Autodesk Inventor part; units mm, degrees
(part 7 of 8)
  spline S913 degree 2 poles (4.9538, -42.7819) (5.0752, -42.7819) (5.2452, -42.6119) (5.2452, -42.4904) knots 0 0 0 1 2 2 2
  line L2980 (4.9538, -42.7819) -> (5.0752, -42.7819) construction
  line L2981 (5.0752, -42.7819) -> (5.2452, -42.6119) construction
  line L2982 (5.2452, -42.6119) -> (5.2452, -42.4904) construction
  line L2983 (5.2452, -42.4904) -> (5.2452, -40.9986)
  spline S914 degree 2 poles (5.2452, -40.9986) (5.2452, -40.8772) (5.0752, -40.7072) (4.9538, -40.7072) knots 0 0 0 1 2 2 2
  line L2984 (5.2452, -40.9986) -> (5.2452, -40.8772) construction
  line L2985 (5.2452, -40.8772) -> (5.0752, -40.7072) construction
  line L2986 (5.0752, -40.7072) -> (4.9538, -40.7072) construction
  line L2987 (4.9538, -40.7072) -> (4.7075, -40.7072)
  spline S915 degree 2 poles (4.7075, -40.7072) (4.5861, -40.7072) (4.4161, -40.8807) (4.4161, -40.9986) knots 0 0 0 1 2 2 2
  line L2988 (4.7075, -40.7072) -> (4.5861, -40.7072) construction
  line L2989 (4.5861, -40.7072) -> (4.4161, -40.8807) construction
  line L2990 (4.4161, -40.8807) -> (4.4161, -40.9986) construction
  line L2991 (4.4161, -40.9986) -> (4.4161, -42.4904)
  spline S916 degree 2 poles (4.4161, -42.4904) (4.4161, -42.6119) (4.5861, -42.7819) (4.7075, -42.7819) knots 0 0 0 1 2 2 2
  line L2992 (4.4161, -42.4904) -> (4.4161, -42.6119) construction
  line L2993 (4.4161, -42.6119) -> (4.5861, -42.7819) construction
  line L2994 (4.5861, -42.7819) -> (4.7075, -42.7819) construction
  line L2995 (4.7075, -42.7819) -> (4.9538, -42.7819)
  spline S917 degree 2 poles (3.9997, -40.9952) (3.9997, -40.7072) (4.4126, -40.2909) (4.7075, -40.2909) knots 0 0 0 1 2 2 2
  line L2996 (3.9997, -40.9952) -> (3.9997, -40.7072) construction
  line L2997 (3.9997, -40.7072) -> (4.4126, -40.2909) construction
  line L2998 (4.4126, -40.2909) -> (4.7075, -40.2909) construction
  line L2999 (4.7075, -40.2909) -> (4.9538, -40.2909)
  spline S918 degree 2 poles (4.9538, -40.2909) (5.2487, -40.2909) (5.6616, -40.7037) (5.6616, -40.9986) knots 0 0 0 1 2 2 2
  line L3000 (4.9538, -40.2909) -> (5.2487, -40.2909) construction
  line L3001 (5.2487, -40.2909) -> (5.6616, -40.7037) construction
  line L3002 (5.6616, -40.7037) -> (5.6616, -40.9986) construction
  line L3003 (5.6616, -40.9986) -> (5.6616, -42.4904)
  spline S919 degree 2 poles (5.6616, -42.4904) (5.6616, -42.7853) (5.2487, -43.1982) (4.9538, -43.1982) knots 0 0 0 1 2 2 2
  line L3004 (5.6616, -42.4904) -> (5.6616, -42.7853) construction
  line L3005 (5.6616, -42.7853) -> (5.2487, -43.1982) construction
  line L3006 (5.2487, -43.1982) -> (4.9538, -43.1982) construction
  line L3007 (4.9538, -43.1982) -> (4.7075, -43.1982)
  spline S920 degree 2 poles (4.7075, -43.1982) (4.4126, -43.1982) (3.9997, -42.7888) (3.9997, -42.4939) knots 0 0 0 1 2 2 2
  line L3008 (4.7075, -43.1982) -> (4.4126, -43.1982) construction
  line L3009 (4.4126, -43.1982) -> (3.9997, -42.7888) construction
  line L3010 (3.9997, -42.7888) -> (3.9997, -42.4939) construction
  spline S921 degree 2 poles (3.5869, -42.99) (3.5869, -43.1982) (3.3787, -43.1982) knots 0 0 0 1 1 1
  line L3011 (3.5869, -42.99) -> (3.5869, -43.1982) construction
  line L3012 (3.5869, -43.1982) -> (3.3787, -43.1982) construction
  spline S922 degree 2 poles (3.3787, -43.1982) (3.1706, -43.1982) (3.1706, -42.99) knots 0 0 0 1 1 1
  line L3013 (3.3787, -43.1982) -> (3.1706, -43.1982) construction
  line L3014 (3.1706, -43.1982) -> (3.1706, -42.99) construction
  line L3015 (3.1706, -42.99) -> (3.1706, -40.499)
  spline S923 degree 2 poles (3.1706, -40.499) (3.1706, -40.2909) (3.3787, -40.2909) knots 0 0 0 1 1 1
  line L3016 (3.1706, -40.499) -> (3.1706, -40.2909) construction
  line L3017 (3.1706, -40.2909) -> (3.3787, -40.2909) construction
  spline S924 degree 2 poles (3.3787, -40.2909) (3.5869, -40.2909) (3.5869, -40.499) knots 0 0 0 1 1 1
  line L3018 (3.3787, -40.2909) -> (3.5869, -40.2909) construction
  line L3019 (3.5869, -40.2909) -> (3.5869, -40.499) construction
  spline S925 degree 2 poles (8.9852, -40.499) (8.9852, -40.2909) (9.1933, -40.2909) knots 0 0 0 1 1 1
  line L3020 (8.9852, -40.499) -> (8.9852, -40.2909) construction
  line L3021 (8.9852, -40.2909) -> (9.1933, -40.2909) construction
  spline S926 degree 2 poles (9.1933, -40.2909) (9.4015, -40.2909) (9.4015, -40.499) knots 0 0 0 1 1 1
  line L3022 (9.1933, -40.2909) -> (9.4015, -40.2909) construction
  line L3023 (9.4015, -40.2909) -> (9.4015, -40.499) construction
  spline S927 degree 2 poles (9.6097, -42.7819) (9.8178, -42.7819) (9.8178, -42.99) knots 0 0 0 1 1 1
  line L3024 (9.6097, -42.7819) -> (9.8178, -42.7819) construction
  line L3025 (9.8178, -42.7819) -> (9.8178, -42.99) construction
  line L3026 (9.8178, -42.99) -> (9.8178, -43.4029)
  spline S928 degree 2 poles (9.8178, -43.4029) (9.8178, -43.611) (9.6097, -43.611) knots 0 0 0 1 1 1
  line L3027 (9.8178, -43.4029) -> (9.8178, -43.611) construction
  line L3028 (9.8178, -43.611) -> (9.6097, -43.611) construction
  spline S929 degree 2 poles (9.6097, -43.611) (9.4015, -43.611) (9.4015, -43.4029) knots 0 0 0 1 1 1
  line L3029 (9.6097, -43.611) -> (9.4015, -43.611) construction
  line L3030 (9.4015, -43.611) -> (9.4015, -43.4029) construction
  spline S930 degree 2 poles (7.3234, -43.1982) (6.9799, -43.1982) (6.4942, -42.7125) (6.4942, -42.369) knots 0 0 0 1 2 2 2
  line L3031 (7.3234, -43.1982) -> (6.9799, -43.1982) construction
  line L3032 (6.9799, -43.1982) -> (6.4942, -42.7125) construction
  line L3033 (6.4942, -42.7125) -> (6.4942, -42.369) construction
  line L3034 (6.4942, -42.369) -> (6.4942, -40.499)
  spline S931 degree 2 poles (6.4942, -40.499) (6.4942, -40.2909) (6.7024, -40.2909) knots 0 0 0 1 1 1
  line L3035 (6.4942, -40.499) -> (6.4942, -40.2909) construction
  line L3036 (6.4942, -40.2909) -> (6.7024, -40.2909) construction
  spline S932 degree 2 poles (6.7024, -40.2909) (6.9105, -40.2909) (6.9105, -40.499) knots 0 0 0 1 1 1
  line L3037 (6.7024, -40.2909) -> (6.9105, -40.2909) construction
  line L3038 (6.9105, -40.2909) -> (6.9105, -40.499) construction
  line L3039 (6.9105, -40.499) -> (6.9105, -42.3655)
  spline S933 degree 2 poles (6.9105, -42.3655) (6.9105, -42.5355) (7.1568, -42.7819) (7.3268, -42.7819) knots 0 0 0 1 2 2 2
  line L3040 (6.9105, -42.3655) -> (6.9105, -42.5355) construction
  line L3041 (6.9105, -42.5355) -> (7.1568, -42.7819) construction
  line L3042 (7.1568, -42.7819) -> (7.3268, -42.7819) construction
  spline S934 degree 2 poles (7.7397, -40.499) (7.7397, -40.2909) (7.9478, -40.2909) knots 0 0 0 1 1 1
  line L3043 (7.7397, -40.499) -> (7.7397, -40.2909) construction
  line L3044 (7.7397, -40.2909) -> (7.9478, -40.2909) construction
  spline S935 degree 2 poles (7.9478, -40.2909) (8.156, -40.2909) (8.156, -40.499) knots 0 0 0 1 1 1
  line L3045 (7.9478, -40.2909) -> (8.156, -40.2909) construction
  line L3046 (8.156, -40.2909) -> (8.156, -40.499) construction
  spline S936 degree 2 poles (-14.1653, -55.9201) (-14.5801, -55.9201) (-15.1811, -55.3275) (-15.1811, -54.9085) knots 0 0 0 1 2 2 2
  line L3047 (-14.1653, -55.9201) -> (-14.5801, -55.9201) construction
  line L3048 (-14.5801, -55.9201) -> (-15.1811, -55.3275) construction
  line L3049 (-15.1811, -55.3275) -> (-15.1811, -54.9085) construction
  line L3050 (-15.1811, -54.9085) -> (-15.1811, -53.3848)
  spline S937 degree 2 poles (-15.1811, -53.3848) (-15.1811, -52.9657) (-14.5801, -52.3732) (-14.1653, -52.3732) knots 0 0 0 1 2 2 2
  line L3051 (-15.1811, -53.3848) -> (-15.1811, -52.9657) construction
  line L3052 (-15.1811, -52.9657) -> (-14.5801, -52.3732) construction
  line L3053 (-14.5801, -52.3732) -> (-14.1653, -52.3732) construction
  line L3054 (-14.1653, -52.3732) -> (-13.4076, -52.3732)
  spline S938 degree 2 poles (-13.4076, -52.3732) (-13.1537, -52.3732) (-13.1537, -52.6271) knots 0 0 0 1 1 1
  line L3055 (-13.4076, -52.3732) -> (-13.1537, -52.3732) construction
  line L3056 (-13.1537, -52.3732) -> (-13.1537, -52.6271) construction
  spline S939 degree 2 poles (-13.1537, -52.6271) (-13.1537, -52.8811) (-13.4076, -52.8811) knots 0 0 0 1 1 1
  line L3057 (-13.1537, -52.6271) -> (-13.1537, -52.8811) construction
  line L3058 (-13.1537, -52.8811) -> (-13.4076, -52.8811) construction
  line L3059 (-13.4076, -52.8811) -> (-14.1653, -52.8811)
  spline S940 degree 2 poles (-14.1653, -52.8811) (-14.3727, -52.8811) (-14.6732, -53.1816) (-14.6732, -53.389) knots 0 0 0 1 2 2 2
  line L3060 (-14.1653, -52.8811) -> (-14.3727, -52.8811) construction
  line L3061 (-14.3727, -52.8811) -> (-14.6732, -53.1816) construction
  line L3062 (-14.6732, -53.1816) -> (-14.6732, -53.389) construction
  line L3063 (-14.6732, -53.389) -> (-14.6732, -54.9043)
  spline S941 degree 2 poles (-14.6732, -54.9043) (-14.6732, -55.1117) (-14.3727, -55.4122) (-14.1653, -55.4122) knots 0 0 0 1 2 2 2
  line L3064 (-14.6732, -54.9043) -> (-14.6732, -55.1117) construction
  line L3065 (-14.6732, -55.1117) -> (-14.3727, -55.4122) construction
  line L3066 (-14.3727, -55.4122) -> (-14.1653, -55.4122) construction
  line L3067 (-14.1653, -55.4122) -> (-13.4076, -55.4122)
  spline S942 degree 2 poles (-13.4076, -55.4122) (-13.1537, -55.4122) (-13.1537, -55.6661) knots 0 0 0 1 1 1
  line L3068 (-13.4076, -55.4122) -> (-13.1537, -55.4122) construction
  line L3069 (-13.1537, -55.4122) -> (-13.1537, -55.6661) construction
  spline S943 degree 2 poles (-13.1537, -55.6661) (-13.1537, -55.9201) (-13.4076, -55.9201) knots 0 0 0 1 1 1
  line L3070 (-13.1537, -55.6661) -> (-13.1537, -55.9201) construction
  line L3071 (-13.1537, -55.9201) -> (-13.4076, -55.9201) construction
  line L3072 (-13.4076, -55.9201) -> (-14.1653, -55.9201)
  spline S944 degree 2 poles (-4.8151, -54.2617) (-5.2315, -54.2617) (-5.2315, -53.8454) knots 0 0 0 1 1 1
  line L3073 (-4.8151, -54.2617) -> (-5.2315, -54.2617) construction
  line L3074 (-5.2315, -54.2617) -> (-5.2315, -53.8454) construction
  spline S945 degree 2 poles (-5.2315, -53.8454) (-5.2315, -53.4291) (-4.8151, -53.4291) knots 0 0 0 1 1 1
  line L3075 (-5.2315, -53.8454) -> (-5.2315, -53.4291) construction
  line L3076 (-5.2315, -53.4291) -> (-4.8151, -53.4291) construction
  line L3077 (-4.8151, -53.4291) -> (-1.4915, -53.4291)
  spline S946 degree 2 poles (-1.4915, -53.4291) (-1.0821, -53.4291) (-1.0821, -53.8454) knots 0 0 0 1 1 1
  line L3078 (-1.4915, -53.4291) -> (-1.0821, -53.4291) construction
  line L3079 (-1.0821, -53.4291) -> (-1.0821, -53.8454) construction
  spline S947 degree 2 poles (-1.0821, -53.8454) (-1.0821, -54.2617) (-1.4915, -54.2617) knots 0 0 0 1 1 1
  line L3080 (-1.0821, -53.8454) -> (-1.0821, -54.2617) construction
  line L3081 (-1.0821, -54.2617) -> (-1.4915, -54.2617) construction
  line L3082 (-1.4915, -54.2617) -> (-4.8151, -54.2617)
  spline S948 degree 2 poles (-18.0718, -61.1463) (-18.0718, -60.9382) (-17.8637, -60.9382) knots 0 0 0 1 1 1
  line L3083 (-18.0718, -61.1463) -> (-18.0718, -60.9382) construction
  line L3084 (-18.0718, -60.9382) -> (-17.8637, -60.9382) construction
  spline S949 degree 2 poles (-17.8637, -60.9382) (-17.6555, -60.9382) (-17.6555, -61.1463) knots 0 0 0 1 1 1
  line L3085 (-17.8637, -60.9382) -> (-17.6555, -60.9382) construction
  line L3086 (-17.6555, -60.9382) -> (-17.6555, -61.1463) construction
  line L3087 (-17.6555, -61.1463) -> (-17.6555, -63.6373)
  spline S950 degree 2 poles (-17.6555, -63.6373) (-17.6555, -63.8455) (-17.8637, -63.8455) knots 0 0 0 1 1 1
  line L3088 (-17.6555, -63.6373) -> (-17.6555, -63.8455) construction
  line L3089 (-17.6555, -63.8455) -> (-17.8637, -63.8455) construction
  spline S951 degree 2 poles (-17.8637, -63.8455) (-18.0718, -63.8455) (-18.0718, -63.6373) knots 0 0 0 1 1 1
  line L3090 (-17.8637, -63.8455) -> (-18.0718, -63.8455) construction
  line L3091 (-18.0718, -63.8455) -> (-18.0718, -63.6373) construction
  spline S952 degree 2 poles (-19.3139, -63.6373) (-19.3139, -63.8455) (-19.522, -63.8455) knots 0 0 0 1 1 1
  line L3092 (-19.3139, -63.6373) -> (-19.3139, -63.8455) construction
  line L3093 (-19.3139, -63.8455) -> (-19.522, -63.8455) construction
  spline S953 degree 2 poles (-19.522, -63.8455) (-19.7302, -63.8455) (-19.7302, -63.6373) knots 0 0 0 1 1 1
  line L3094 (-19.522, -63.8455) -> (-19.7302, -63.8455) construction
  line L3095 (-19.7302, -63.8455) -> (-19.7302, -63.6373) construction
  line L3096 (-19.7302, -63.6373) -> (-19.7302, -61.1463)
  spline S954 degree 2 poles (-19.7302, -61.1463) (-19.7302, -60.9382) (-19.522, -60.9382) knots 0 0 0 1 1 1
  line L3097 (-19.7302, -61.1463) -> (-19.7302, -60.9382) construction
  line L3098 (-19.7302, -60.9382) -> (-19.522, -60.9382) construction
  spline S955 degree 2 poles (-19.522, -60.9382) (-19.3139, -60.9382) (-19.3139, -61.1463) knots 0 0 0 1 1 1
  line L3099 (-19.522, -60.9382) -> (-19.3139, -60.9382) construction
  line L3100 (-19.3139, -60.9382) -> (-19.3139, -61.1463) construction
  spline S956 degree 2 poles (-9.1418, -63.8455) (-9.3499, -63.8455) (-9.3499, -63.6373) knots 0 0 0 1 1 1
  line L3101 (-9.1418, -63.8455) -> (-9.3499, -63.8455) construction
  line L3102 (-9.3499, -63.8455) -> (-9.3499, -63.6373) construction
  spline S957 degree 2 poles (-10.6058, -63.7032) (-10.6509, -63.8455) (-10.7897, -63.8455) knots 0 0 0 1 1 1
  line L3103 (-10.6058, -63.7032) -> (-10.6509, -63.8455) construction
  line L3104 (-10.6509, -63.8455) -> (-10.7897, -63.8455) construction
  spline S958 degree 2 poles (-10.7897, -63.8455) (-11.0083, -63.8455) (-11.0083, -63.6477) knots 0 0 0 1 1 1
  line L3105 (-10.7897, -63.8455) -> (-11.0083, -63.8455) construction
  line L3106 (-11.0083, -63.8455) -> (-11.0083, -63.6477) construction
  spline S959 degree 2 poles (-11.0083, -63.6477) (-11.0083, -63.6096) (-10.9944, -63.5714) knots 0 0 0 1 1 1
  line L3107 (-11.0083, -63.6477) -> (-11.0083, -63.6096) construction
  line L3108 (-11.0083, -63.6096) -> (-10.9944, -63.5714) construction
  line L3109 (-10.9944, -63.5714) -> (-10.1722, -61.0804)
  spline S960 degree 2 poles (-10.1722, -61.0804) (-10.1271, -60.9382) (-9.9779, -60.9382) knots 0 0 0 1 1 1
  line L3110 (-10.1722, -61.0804) -> (-10.1271, -60.9382) construction
  line L3111 (-10.1271, -60.9382) -> (-9.9779, -60.9382) construction
  line L3112 (-9.9779, -60.9382) -> (-9.1418, -60.9382)
  spline S961 degree 2 poles (-9.1418, -60.9382) (-8.9336, -60.9382) (-8.9336, -61.1463) knots 0 0 0 1 1 1
  line L3113 (-9.1418, -60.9382) -> (-8.9336, -60.9382) construction
  line L3114 (-8.9336, -60.9382) -> (-8.9336, -61.1463) construction
  line L3115 (-8.9336, -61.1463) -> (-8.9336, -63.6373)
  spline S962 degree 2 poles (-8.9336, -63.6373) (-8.9336, -63.8455) (-9.1418, -63.8455) knots 0 0 0 1 1 1
  line L3116 (-8.9336, -63.6373) -> (-8.9336, -63.8455) construction
  line L3117 (-8.9336, -63.8455) -> (-9.1418, -63.8455) construction
  spline S963 degree 2 poles (1.8629, -61.1463) (1.8629, -60.9382) (2.0711, -60.9382) knots 0 0 0 1 1 1
  line L3118 (1.8629, -61.1463) -> (1.8629, -60.9382) construction
  line L3119 (1.8629, -60.9382) -> (2.0711, -60.9382) construction
  spline S964 degree 2 poles (2.0711, -60.9382) (2.2793, -60.9382) (2.2793, -61.1463) knots 0 0 0 1 1 1
  line L3120 (2.0711, -60.9382) -> (2.2793, -60.9382) construction
  line L3121 (2.2793, -60.9382) -> (2.2793, -61.1463) construction
  line L3122 (2.2793, -61.1463) -> (2.2793, -63.6373)
  spline S965 degree 2 poles (2.2793, -63.6373) (2.2793, -63.8455) (2.0711, -63.8455) knots 0 0 0 1 1 1
  line L3123 (2.2793, -63.6373) -> (2.2793, -63.8455) construction
  line L3124 (2.2793, -63.8455) -> (2.0711, -63.8455) construction
  spline S966 degree 2 poles (2.0711, -63.8455) (1.8629, -63.8455) (1.8629, -63.6373) knots 0 0 0 1 1 1
  line L3125 (2.0711, -63.8455) -> (1.8629, -63.8455) construction
  line L3126 (1.8629, -63.8455) -> (1.8629, -63.6373) construction
  spline S967 degree 2 poles (0.6209, -63.6373) (0.6209, -63.8455) (0.4128, -63.8455) knots 0 0 0 1 1 1
  line L3127 (0.6209, -63.6373) -> (0.6209, -63.8455) construction
  line L3128 (0.6209, -63.8455) -> (0.4128, -63.8455) construction
  spline S968 degree 2 poles (0.4128, -63.8455) (0.2046, -63.8455) (0.2046, -63.6373) knots 0 0 0 1 1 1
  line L3129 (0.4128, -63.8455) -> (0.2046, -63.8455) construction
  line L3130 (0.2046, -63.8455) -> (0.2046, -63.6373) construction
  line L3131 (0.2046, -63.6373) -> (0.2046, -61.1463)
  spline S969 degree 2 poles (0.2046, -61.1463) (0.2046, -60.9382) (0.4128, -60.9382) knots 0 0 0 1 1 1
  line L3132 (0.2046, -61.1463) -> (0.2046, -60.9382) construction
  line L3133 (0.2046, -60.9382) -> (0.4128, -60.9382) construction
  spline S970 degree 2 poles (0.4128, -60.9382) (0.6209, -60.9382) (0.6209, -61.1463) knots 0 0 0 1 1 1
  line L3134 (0.4128, -60.9382) -> (0.6209, -60.9382) construction
  line L3135 (0.6209, -60.9382) -> (0.6209, -61.1463) construction
  spline S971 degree 2 poles (10.172, -63.4292) (10.342, -63.4292) (10.5848, -63.1828) (10.5848, -63.0128) knots 0 0 0 1 2 2 2
  line L3136 (10.172, -63.4292) -> (10.342, -63.4292) construction
  line L3137 (10.342, -63.4292) -> (10.5848, -63.1828) construction
  line L3138 (10.5848, -63.1828) -> (10.5848, -63.0128) construction
  line L3139 (10.5848, -63.0128) -> (10.5848, -61.7708)
  spline S972 degree 2 poles (10.5848, -61.7708) (10.5848, -61.6008) (10.342, -61.3545) (10.172, -61.3545) knots 0 0 0 1 2 2 2
  line L3140 (10.5848, -61.7708) -> (10.5848, -61.6008) construction
  line L3141 (10.5848, -61.6008) -> (10.342, -61.3545) construction
  line L3142 (10.342, -61.3545) -> (10.172, -61.3545) construction
  spline S973 degree 2 poles (9.3428, -64.8828) (9.3428, -65.091) (9.1347, -65.091) knots 0 0 0 1 1 1
  line L3143 (9.3428, -64.8828) -> (9.3428, -65.091) construction
  line L3144 (9.3428, -65.091) -> (9.1347, -65.091) construction
  spline S974 degree 2 poles (9.1347, -65.091) (8.9265, -65.091) (8.9265, -64.8828) knots 0 0 0 1 1 1
  line L3145 (9.1347, -65.091) -> (8.9265, -65.091) construction
  line L3146 (8.9265, -65.091) -> (8.9265, -64.8828) construction
  line L3147 (8.9265, -64.8828) -> (8.9265, -61.1463)
  spline S975 degree 2 poles (8.9265, -61.1463) (8.9265, -60.9382) (9.1347, -60.9382) knots 0 0 0 1 1 1
  line L3148 (8.9265, -61.1463) -> (8.9265, -60.9382) construction
  line L3149 (8.9265, -60.9382) -> (9.1347, -60.9382) construction
  line L3150 (9.1347, -60.9382) -> (10.172, -60.9382)
  spline S976 degree 2 poles (10.172, -60.9382) (10.5155, -60.9382) (11.0012, -61.4239) (11.0012, -61.7674) knots 0 0 0 1 2 2 2
  line L3151 (10.172, -60.9382) -> (10.5155, -60.9382) construction
  line L3152 (10.5155, -60.9382) -> (11.0012, -61.4239) construction
  line L3153 (11.0012, -61.4239) -> (11.0012, -61.7674) construction
  line L3154 (11.0012, -61.7674) -> (11.0012, -63.0163)
  spline S977 degree 2 poles (11.0012, -63.0163) (11.0012, -63.3598) (10.5155, -63.8455) (10.172, -63.8455) knots 0 0 0 1 2 2 2
  line L3155 (11.0012, -63.0163) -> (11.0012, -63.3598) construction
  line L3156 (11.0012, -63.3598) -> (10.5155, -63.8455) construction
  line L3157 (10.5155, -63.8455) -> (10.172, -63.8455) construction
  spline S978 degree 2 poles (13.0793, -63.4292) (13.2493, -63.4292) (13.4921, -63.1828) (13.4921, -63.0128) knots 0 0 0 1 2 2 2
  line L3158 (13.0793, -63.4292) -> (13.2493, -63.4292) construction
  line L3159 (13.2493, -63.4292) -> (13.4921, -63.1828) construction
  line L3160 (13.4921, -63.1828) -> (13.4921, -63.0128) construction
  spline S979 degree 2 poles (12.663, -61.3545) (12.493, -61.3545) (12.2501, -61.6008) (12.2501, -61.7708) knots 0 0 0 1 2 2 2
  line L3161 (12.663, -61.3545) -> (12.493, -61.3545) construction
  line L3162 (12.493, -61.3545) -> (12.2501, -61.6008) construction
  line L3163 (12.2501, -61.6008) -> (12.2501, -61.7708) construction
  line L3164 (12.2501, -61.7708) -> (12.2501, -63.0128)
  spline S980 degree 2 poles (12.2501, -63.0128) (12.2501, -63.1828) (12.493, -63.4292) (12.663, -63.4292) knots 0 0 0 1 2 2 2
  line L3165 (12.2501, -63.0128) -> (12.2501, -63.1828) construction
  line L3166 (12.2501, -63.1828) -> (12.493, -63.4292) construction
  line L3167 (12.493, -63.4292) -> (12.663, -63.4292) construction
  line L3168 (12.663, -63.4292) -> (13.0793, -63.4292)
  line L3169 (13.0793, -63.8455) -> (12.663, -63.8455)
  spline S981 degree 2 poles (12.663, -63.8455) (12.323, -63.8455) (11.8338, -63.3598) (11.8338, -63.0163) knots 0 0 0 1 2 2 2
  line L3170 (12.663, -63.8455) -> (12.323, -63.8455) construction
  line L3171 (12.323, -63.8455) -> (11.8338, -63.3598) construction
  line L3172 (11.8338, -63.3598) -> (11.8338, -63.0163) construction
  line L3173 (11.8338, -63.0163) -> (11.8338, -61.7674)
  spline S982 degree 2 poles (11.8338, -61.7674) (11.8338, -61.4239) (12.323, -60.9382) (12.663, -60.9382) knots 0 0 0 1 2 2 2
  line L3174 (11.8338, -61.7674) -> (11.8338, -61.4239) construction
  line L3175 (11.8338, -61.4239) -> (12.323, -60.9382) construction
  line L3176 (12.323, -60.9382) -> (12.663, -60.9382) construction
  line L3177 (12.663, -60.9382) -> (13.7003, -60.9382)
  spline S983 degree 2 poles (13.7003, -60.9382) (13.9085, -60.9382) (13.9085, -61.1463) knots 0 0 0 1 1 1
  line L3178 (13.7003, -60.9382) -> (13.9085, -60.9382) construction
  line L3179 (13.9085, -60.9382) -> (13.9085, -61.1463) construction
  line L3180 (13.9085, -61.1463) -> (13.9085, -63.0094)
  spline S984 degree 2 poles (13.9085, -63.0094) (13.9085, -63.3216) (14.1999, -63.4465) knots 0 0 0 1 1 1
  line L3181 (13.9085, -63.0094) -> (13.9085, -63.3216) construction
  line L3182 (13.9085, -63.3216) -> (14.1999, -63.4465) construction
  spline S985 degree 2 poles (14.1999, -63.4465) (14.3283, -63.4985) (14.3283, -63.6304) knots 0 0 0 1 1 1
  line L3183 (14.1999, -63.4465) -> (14.3283, -63.4985) construction
  line L3184 (14.3283, -63.4985) -> (14.3283, -63.6304) construction
  spline S986 degree 2 poles (14.3283, -63.6304) (14.3283, -63.7171) (14.2103, -63.849) (14.1236, -63.849) knots 0 0 0 1 2 2 2
  line L3185 (14.3283, -63.6304) -> (14.3283, -63.7171) construction
  line L3186 (14.3283, -63.7171) -> (14.2103, -63.849) construction
  line L3187 (14.2103, -63.849) -> (14.1236, -63.849) construction
  spline S987 degree 2 poles (14.1236, -63.849) (14.0785, -63.849) (14.0334, -63.8281) knots 0 0 0 1 1 1
  line L3188 (14.1236, -63.849) -> (14.0785, -63.849) construction
  line L3189 (14.0785, -63.849) -> (14.0334, -63.8281) construction
  spline S988 degree 2 poles (14.0334, -63.8281) (13.8252, -63.7379) (13.6968, -63.5714) knots 0 0 0 1 1 1
  line L3190 (14.0334, -63.8281) -> (13.8252, -63.7379) construction
  line L3191 (13.8252, -63.7379) -> (13.6968, -63.5714) construction
  spline S989 degree 2 poles (13.6968, -63.5714) (13.447, -63.8455) (13.0793, -63.8455) knots 0 0 0 1 1 1
  line L3192 (13.6968, -63.5714) -> (13.447, -63.8455) construction
  line L3193 (13.447, -63.8455) -> (13.0793, -63.8455) construction
  line L3194 (15.1574, -60.4386) -> (15.1574, -61.0839)
  spline S990 degree 2 poles (15.1574, -61.0839) (15.3205, -60.9798) (15.5703, -60.7959) knots 0 0 0 1 1 1
  line L3195 (15.1574, -61.0839) -> (15.3205, -60.9798) construction
  line L3196 (15.3205, -60.9798) -> (15.5703, -60.7959) construction
  spline S991 degree 2 poles (15.5703, -60.7959) (15.8201, -60.5947) (15.8201, -60.4386) knots 0 0 0 1 1 1
  line L3197 (15.5703, -60.7959) -> (15.8201, -60.5947) construction
  line L3198 (15.8201, -60.5947) -> (15.8201, -60.4386) construction
  spline S992 degree 2 poles (15.8201, -60.4386) (15.8201, -60.279) (15.716, -60.1888) knots 0 0 0 1 1 1
  line L3199 (15.8201, -60.4386) -> (15.8201, -60.279) construction
  line L3200 (15.8201, -60.279) -> (15.716, -60.1888) construction
  spline S993 degree 2 poles (15.716, -60.1888) (15.6223, -60.109) (15.4905, -60.109) knots 0 0 0 1 1 1
  line L3201 (15.716, -60.1888) -> (15.6223, -60.109) construction
  line L3202 (15.6223, -60.109) -> (15.4905, -60.109) construction
  spline S994 degree 2 poles (15.4905, -60.109) (15.3517, -60.109) (15.2615, -60.1888) knots 0 0 0 1 1 1
  line L3203 (15.4905, -60.109) -> (15.3517, -60.109) construction
  line L3204 (15.3517, -60.109) -> (15.2615, -60.1888) construction
  spline S995 degree 2 poles (15.2615, -60.1888) (15.1574, -60.279) (15.1574, -60.4386) knots 0 0 0 1 1 1
  line L3205 (15.2615, -60.1888) -> (15.1574, -60.279) construction
  line L3206 (15.1574, -60.279) -> (15.1574, -60.4386) construction
  spline S996 degree 2 poles (15.9866, -63.4292) (16.1566, -63.4292) (16.3994, -63.1828) (16.3994, -63.0128) knots 0 0 0 1 2 2 2
  line L3207 (15.9866, -63.4292) -> (16.1566, -63.4292) construction
  line L3208 (16.1566, -63.4292) -> (16.3994, -63.1828) construction
  line L3209 (16.3994, -63.1828) -> (16.3994, -63.0128) construction
  line L3210 (16.3994, -63.0128) -> (16.3994, -61.7674)
  spline S997 degree 2 poles (16.3994, -61.7674) (16.3994, -61.5974) (16.1566, -61.351) (15.9866, -61.351) knots 0 0 0 1 2 2 2
  line L3211 (16.3994, -61.7674) -> (16.3994, -61.5974) construction
  line L3212 (16.3994, -61.5974) -> (16.1566, -61.351) construction
  line L3213 (16.1566, -61.351) -> (15.9866, -61.351) construction
  line L3214 (15.9866, -61.351) -> (15.5703, -61.351)
  spline S998 degree 2 poles (15.5703, -61.351) (15.4003, -61.351) (15.1574, -61.5974) (15.1574, -61.7674) knots 0 0 0 1 2 2 2
  line L3215 (15.5703, -61.351) -> (15.4003, -61.351) construction
  line L3216 (15.4003, -61.351) -> (15.1574, -61.5974) construction
  line L3217 (15.1574, -61.5974) -> (15.1574, -61.7674) construction
  line L3218 (15.1574, -61.7674) -> (15.1574, -63.0128)
  spline S999 degree 2 poles (15.1574, -63.0128) (15.1574, -63.1828) (15.4003, -63.4292) (15.5703, -63.4292) knots 0 0 0 1 2 2 2
  line L3219 (15.1574, -63.0128) -> (15.1574, -63.1828) construction
  line L3220 (15.1574, -63.1828) -> (15.4003, -63.4292) construction
  line L3221 (15.4003, -63.4292) -> (15.5703, -63.4292) construction
  line L3222 (15.5703, -63.4292) -> (15.9866, -63.4292)
  spline S1000 degree 2 poles (16.6111, -61.188) (16.8158, -61.4065) (16.8158, -61.7674) knots 0 0 0 1 1 1
  line L3223 (16.6111, -61.188) -> (16.8158, -61.4065) construction
  line L3224 (16.8158, -61.4065) -> (16.8158, -61.7674) construction
  line L3225 (16.8158, -61.7674) -> (16.8158, -63.0163)
  spline S1001 degree 2 poles (16.8158, -63.0163) (16.8158, -63.3598) (16.3301, -63.8455) (15.9866, -63.8455) knots 0 0 0 1 2 2 2
  line L3226 (16.8158, -63.0163) -> (16.8158, -63.3598) construction
  line L3227 (16.8158, -63.3598) -> (16.3301, -63.8455) construction
  line L3228 (16.3301, -63.8455) -> (15.9866, -63.8455) construction
  line L3229 (15.9866, -63.8455) -> (15.5703, -63.8455)
  spline S1002 degree 2 poles (15.5703, -63.8455) (15.2303, -63.8455) (14.7411, -63.3598) (14.7411, -63.0163) knots 0 0 0 1 2 2 2
  line L3230 (15.5703, -63.8455) -> (15.2303, -63.8455) construction
  line L3231 (15.2303, -63.8455) -> (14.7411, -63.3598) construction
  line L3232 (14.7411, -63.3598) -> (14.7411, -63.0163) construction
  line L3233 (14.7411, -63.0163) -> (14.7411, -60.4386)
  spline S1003 degree 2 poles (14.7411, -60.4386) (14.7411, -60.0882) (14.9735, -59.88) knots 0 0 0 1 1 1
  line L3234 (14.7411, -60.4386) -> (14.7411, -60.0882) construction
  line L3235 (14.7411, -60.0882) -> (14.9735, -59.88) construction
  spline S1004 degree 2 poles (14.9735, -59.88) (15.1852, -59.6927) (15.4939, -59.6927) knots 0 0 0 1 1 1
  line L3236 (14.9735, -59.88) -> (15.1852, -59.6927) construction
  line L3237 (15.1852, -59.6927) -> (15.4939, -59.6927) construction
  spline S1005 degree 2 poles (15.4939, -59.6927) (15.7958, -59.6927) (16.0039, -59.8766) knots 0 0 0 1 1 1
  line L3238 (15.4939, -59.6927) -> (15.7958, -59.6927) construction
  line L3239 (15.7958, -59.6927) -> (16.0039, -59.8766) construction
  spline S1006 degree 2 poles (16.0039, -59.8766) (16.2364, -60.0847) (16.2364, -60.4351) knots 0 0 0 1 1 1
  line L3240 (16.0039, -59.8766) -> (16.2364, -60.0847) construction
  line L3241 (16.2364, -60.0847) -> (16.2364, -60.4351) construction
  spline S1007 degree 2 poles (16.2364, -60.4351) (16.2364, -60.7855) (15.9866, -60.9521) knots 0 0 0 1 1 1
  line L3242 (16.2364, -60.4351) -> (16.2364, -60.7855) construction
  line L3243 (16.2364, -60.7855) -> (15.9866, -60.9521) construction
  spline S1008 degree 2 poles (15.9866, -60.9521) (16.389, -60.9521) (16.6111, -61.188) knots 0 0 0 1 1 1
  line L3244 (15.9866, -60.9521) -> (16.389, -60.9521) construction
  line L3245 (16.389, -60.9521) -> (16.6111, -61.188) construction
  spline S1009 degree 2 poles (20.7639, -63.4292) (20.972, -63.4292) (20.972, -63.6373) knots 0 0 0 1 1 1
  line L3246 (20.7639, -63.4292) -> (20.972, -63.4292) construction
  line L3247 (20.972, -63.4292) -> (20.972, -63.6373) construction
  spline S1010 degree 2 poles (20.972, -63.6373) (20.972, -63.8455) (20.7639, -63.8455) knots 0 0 0 1 1 1
  line L3248 (20.972, -63.6373) -> (20.972, -63.8455) construction
  line L3249 (20.972, -63.8455) -> (20.7639, -63.8455) construction
  spline S1011 degree 2 poles (20.7639, -63.8455) (20.5557, -63.8455) (20.5557, -63.6373) knots 0 0 0 1 1 1
  line L3250 (20.7639, -63.8455) -> (20.5557, -63.8455) construction
  line L3251 (20.5557, -63.8455) -> (20.5557, -63.6373) construction
  spline S1012 degree 2 poles (20.5557, -63.6373) (20.5557, -63.4292) (20.7639, -63.4292) knots 0 0 0 1 1 1
  line L3252 (20.5557, -63.6373) -> (20.5557, -63.4292) construction
  line L3253 (20.5557, -63.4292) -> (20.7639, -63.4292) construction
  spline S1013 degree 2 poles (-8.0227, 45.6499) (-7.8284, 45.6499) (-7.7139, 45.7783) knots 0 0 0 1 1 1
  line L3254 (-8.0227, 45.6499) -> (-7.8284, 45.6499) construction
  line L3255 (-7.8284, 45.6499) -> (-7.7139, 45.7783) construction
  spline S1014 degree 2 poles (-7.7139, 45.7783) (-7.6098, 45.8962) (-7.6098, 46.0662) knots 0 0 0 1 1 1
  line L3256 (-7.7139, 45.7783) -> (-7.6098, 45.8962) construction
  line L3257 (-7.6098, 45.8962) -> (-7.6098, 46.0662) construction
  spline S1015 degree 2 poles (-7.6098, 46.0662) (-7.6098, 46.2362) (-7.7139, 46.3507) knots 0 0 0 1 1 1
  line L3258 (-7.6098, 46.0662) -> (-7.6098, 46.2362) construction
  line L3259 (-7.6098, 46.2362) -> (-7.7139, 46.3507) construction
  spline S1016 degree 2 poles (-7.7139, 46.3507) (-7.8284, 46.4791) (-8.0227, 46.4791) knots 0 0 0 1 1 1
  line L3260 (-7.7139, 46.3507) -> (-7.8284, 46.4791) construction
  line L3261 (-7.8284, 46.4791) -> (-8.0227, 46.4791) construction
  spline S1017 degree 2 poles (-8.0227, 46.8954) (-7.6272, 46.8954) (-7.4017, 46.6352) knots 0 0 0 1 1 1
  line L3262 (-8.0227, 46.8954) -> (-7.6272, 46.8954) construction
  line L3263 (-7.6272, 46.8954) -> (-7.4017, 46.6352) construction
  spline S1018 degree 2 poles (-7.4017, 46.6352) (-7.1935, 46.4028) (-7.1935, 46.0662) knots 0 0 0 1 1 1
  line L3264 (-7.4017, 46.6352) -> (-7.1935, 46.4028) construction
  line L3265 (-7.1935, 46.4028) -> (-7.1935, 46.0662) construction
  spline S1019 degree 2 poles (-7.1935, 46.0662) (-7.1935, 45.7297) (-7.4017, 45.4903) knots 0 0 0 1 1 1
  line L3266 (-7.1935, 46.0662) -> (-7.1935, 45.7297) construction
  line L3267 (-7.1935, 45.7297) -> (-7.4017, 45.4903) construction
  spline S1020 degree 2 poles (-7.4017, 45.4903) (-7.6307, 45.2336) (-8.0227, 45.2336) knots 0 0 0 1 1 1
  line L3268 (-7.4017, 45.4903) -> (-7.6307, 45.2336) construction
  line L3269 (-7.6307, 45.2336) -> (-8.0227, 45.2336) construction
  line L3270 (-8.0227, 45.2336) -> (-9.06, 45.2336)
  spline S1021 degree 2 poles (-9.06, 45.2336) (-9.2682, 45.2336) (-9.2682, 45.4417) knots 0 0 0 1 1 1
  line L3271 (-9.06, 45.2336) -> (-9.2682, 45.2336) construction
  line L3272 (-9.2682, 45.2336) -> (-9.2682, 45.4417) construction
  line L3273 (-9.2682, 45.4417) -> (-9.2682, 47.9327)
  spline S1022 degree 2 poles (-9.2682, 47.9327) (-9.2682, 48.1409) (-9.06, 48.1409) knots 0 0 0 1 1 1
  line L3274 (-9.2682, 47.9327) -> (-9.2682, 48.1409) construction
  line L3275 (-9.2682, 48.1409) -> (-9.06, 48.1409) construction
  spline S1023 degree 2 poles (-9.06, 48.1409) (-8.8519, 48.1409) (-8.8519, 47.9327) knots 0 0 0 1 1 1
  line L3276 (-9.06, 48.1409) -> (-8.8519, 48.1409) construction
  line L3277 (-8.8519, 48.1409) -> (-8.8519, 47.9327) construction
  line L3278 (-17.3656, 48.6405) -> (-17.3656, 47.9952)
  spline S1024 degree 2 poles (-17.3656, 47.9952) (-17.2025, 48.0993) (-16.9528, 48.2831) knots 0 0 0 1 1 1
  line L3279 (-17.3656, 47.9952) -> (-17.2025, 48.0993) construction
  line L3280 (-17.2025, 48.0993) -> (-16.9528, 48.2831) construction
  spline S1025 degree 2 poles (-16.9528, 48.2831) (-16.703, 48.4844) (-16.703, 48.6405) knots 0 0 0 1 1 1
  line L3281 (-16.9528, 48.2831) -> (-16.703, 48.4844) construction
  line L3282 (-16.703, 48.4844) -> (-16.703, 48.6405) construction
  spline S1026 degree 2 poles (-16.703, 48.6405) (-16.703, 48.8001) (-16.807, 48.8903) knots 0 0 0 1 1 1
  line L3283 (-16.703, 48.6405) -> (-16.703, 48.8001) construction
  line L3284 (-16.703, 48.8001) -> (-16.807, 48.8903) construction
  spline S1027 degree 2 poles (-16.807, 48.8903) (-16.9007, 48.9701) (-17.0326, 48.9701) knots 0 0 0 1 1 1
  line L3285 (-16.807, 48.8903) -> (-16.9007, 48.9701) construction
  line L3286 (-16.9007, 48.9701) -> (-17.0326, 48.9701) construction
  spline S1028 degree 2 poles (-17.0326, 48.9701) (-17.1713, 48.9701) (-17.2615, 48.8903) knots 0 0 0 1 1 1
  line L3287 (-17.0326, 48.9701) -> (-17.1713, 48.9701) construction
  line L3288 (-17.1713, 48.9701) -> (-17.2615, 48.8903) construction
  spline S1029 degree 2 poles (-17.2615, 48.8903) (-17.3656, 48.8001) (-17.3656, 48.6405) knots 0 0 0 1 1 1
  line L3289 (-17.2615, 48.8903) -> (-17.3656, 48.8001) construction
  line L3290 (-17.3656, 48.8001) -> (-17.3656, 48.6405) construction
  spline S1030 degree 2 poles (-16.5364, 45.6499) (-16.3664, 45.6499) (-16.1236, 45.8962) (-16.1236, 46.0662) knots 0 0 0 1 2 2 2
  line L3291 (-16.5364, 45.6499) -> (-16.3664, 45.6499) construction
  line L3292 (-16.3664, 45.6499) -> (-16.1236, 45.8962) construction
  line L3293 (-16.1236, 45.8962) -> (-16.1236, 46.0662) construction
  line L3294 (-16.1236, 46.0662) -> (-16.1236, 47.3117)
  spline S1031 degree 2 poles (-16.1236, 47.3117) (-16.1236, 47.4817) (-16.3664, 47.728) (-16.5364, 47.728) knots 0 0 0 1 2 2 2
  line L3295 (-16.1236, 47.3117) -> (-16.1236, 47.4817) construction
  line L3296 (-16.1236, 47.4817) -> (-16.3664, 47.728) construction
  line L3297 (-16.3664, 47.728) -> (-16.5364, 47.728) construction
  line L3298 (-16.5364, 47.728) -> (-16.9528, 47.728)
  spline S1032 degree 2 poles (-16.9528, 47.728) (-17.1228, 47.728) (-17.3656, 47.4817) (-17.3656, 47.3117) knots 0 0 0 1 2 2 2
  line L3299 (-16.9528, 47.728) -> (-17.1228, 47.728) construction
  line L3300 (-17.1228, 47.728) -> (-17.3656, 47.4817) construction
  line L3301 (-17.3656, 47.4817) -> (-17.3656, 47.3117) construction
  line L3302 (-17.3656, 47.3117) -> (-17.3656, 46.0662)
  spline S1033 degree 2 poles (-17.3656, 46.0662) (-17.3656, 45.8962) (-17.1228, 45.6499) (-16.9528, 45.6499) knots 0 0 0 1 2 2 2
  line L3303 (-17.3656, 46.0662) -> (-17.3656, 45.8962) construction
  line L3304 (-17.3656, 45.8962) -> (-17.1228, 45.6499) construction
  line L3305 (-17.1228, 45.6499) -> (-16.9528, 45.6499) construction
  line L3306 (-16.9528, 45.6499) -> (-16.5364, 45.6499)
  spline S1034 degree 2 poles (-15.912, 47.8911) (-15.7073, 47.6725) (-15.7073, 47.3117) knots 0 0 0 1 1 1
  line L3307 (-15.912, 47.8911) -> (-15.7073, 47.6725) construction
  line L3308 (-15.7073, 47.6725) -> (-15.7073, 47.3117) construction
  line L3309 (-15.7073, 47.3117) -> (-15.7073, 46.0628)
  spline S1035 degree 2 poles (-15.7073, 46.0628) (-15.7073, 45.7193) (-16.193, 45.2336) (-16.5364, 45.2336) knots 0 0 0 1 2 2 2
  line L3310 (-15.7073, 46.0628) -> (-15.7073, 45.7193) construction
  line L3311 (-15.7073, 45.7193) -> (-16.193, 45.2336) construction
  line L3312 (-16.193, 45.2336) -> (-16.5364, 45.2336) construction
  line L3313 (-16.5364, 45.2336) -> (-16.9528, 45.2336)
  spline S1036 degree 2 poles (-16.9528, 45.2336) (-17.2927, 45.2336) (-17.7819, 45.7193) (-17.7819, 46.0628) knots 0 0 0 1 2 2 2
  line L3314 (-16.9528, 45.2336) -> (-17.2927, 45.2336) construction
  line L3315 (-17.2927, 45.2336) -> (-17.7819, 45.7193) construction
  line L3316 (-17.7819, 45.7193) -> (-17.7819, 46.0628) construction
  line L3317 (-17.7819, 46.0628) -> (-17.7819, 48.6405)
  spline S1037 degree 2 poles (-17.7819, 48.6405) (-17.7819, 48.9909) (-17.5495, 49.199) knots 0 0 0 1 1 1
  line L3318 (-17.7819, 48.6405) -> (-17.7819, 48.9909) construction
  line L3319 (-17.7819, 48.9909) -> (-17.5495, 49.199) construction
  spline S1038 degree 2 poles (-17.5495, 49.199) (-17.3379, 49.3864) (-17.0291, 49.3864) knots 0 0 0 1 1 1
  line L3320 (-17.5495, 49.199) -> (-17.3379, 49.3864) construction
  line L3321 (-17.3379, 49.3864) -> (-17.0291, 49.3864) construction
  spline S1039 degree 2 poles (-17.0291, 49.3864) (-16.7272, 49.3864) (-16.5191, 49.2025) knots 0 0 0 1 1 1
  line L3322 (-17.0291, 49.3864) -> (-16.7272, 49.3864) construction
  line L3323 (-16.7272, 49.3864) -> (-16.5191, 49.2025) construction
  spline S1040 degree 2 poles (-16.5191, 49.2025) (-16.2866, 48.9943) (-16.2866, 48.6439) knots 0 0 0 1 1 1
  line L3324 (-16.5191, 49.2025) -> (-16.2866, 48.9943) construction
  line L3325 (-16.2866, 48.9943) -> (-16.2866, 48.6439) construction
  spline S1041 degree 2 poles (-16.2866, 48.6439) (-16.2866, 48.2935) (-16.5364, 48.127) knots 0 0 0 1 1 1
  line L3326 (-16.2866, 48.6439) -> (-16.2866, 48.2935) construction
  line L3327 (-16.2866, 48.2935) -> (-16.5364, 48.127) construction
  spline S1042 degree 2 poles (-16.5364, 48.127) (-16.134, 48.127) (-15.912, 47.8911) knots 0 0 0 1 1 1
  line L3328 (-16.5364, 48.127) -> (-16.134, 48.127) construction
  line L3329 (-16.134, 48.127) -> (-15.912, 47.8911) construction
  spline S1043 degree 2 poles (-19.4403, 45.2336) (-19.7803, 45.2336) (-20.2729, 45.7193) (-20.2729, 46.0628) knots 0 0 0 1 2 2 2
  line L3330 (-19.4403, 45.2336) -> (-19.7803, 45.2336) construction
  line L3331 (-19.7803, 45.2336) -> (-20.2729, 45.7193) construction
  line L3332 (-20.2729, 45.7193) -> (-20.2729, 46.0628) construction
  line L3333 (-20.2729, 46.0628) -> (-20.2729, 47.3117)
  spline S1044 degree 2 poles (-20.2729, 47.3117) (-20.2729, 47.6552) (-19.7803, 48.1409) (-19.4403, 48.1409) knots 0 0 0 1 2 2 2
  line L3334 (-20.2729, 47.3117) -> (-20.2729, 47.6552) construction
  line L3335 (-20.2729, 47.6552) -> (-19.7803, 48.1409) construction
  line L3336 (-19.7803, 48.1409) -> (-19.4403, 48.1409) construction
  line L3337 (-19.4403, 48.1409) -> (-18.8193, 48.1409)
  spline S1045 degree 2 poles (-18.8193, 48.1409) (-18.6111, 48.1409) (-18.6111, 47.9327) knots 0 0 0 1 1 1
  line L3338 (-18.8193, 48.1409) -> (-18.6111, 48.1409) construction
  line L3339 (-18.6111, 48.1409) -> (-18.6111, 47.9327) construction
  spline S1046 degree 2 poles (-18.6111, 47.9327) (-18.6111, 47.7246) (-18.8193, 47.7246) knots 0 0 0 1 1 1
  line L3340 (-18.6111, 47.9327) -> (-18.6111, 47.7246) construction
  line L3341 (-18.6111, 47.7246) -> (-18.8193, 47.7246) construction
  line L3342 (-18.8193, 47.7246) -> (-19.4403, 47.7246)
  spline S1047 degree 2 poles (-19.4403, 47.7246) (-19.6103, 47.7246) (-19.8566, 47.4782) (-19.8566, 47.3082) knots 0 0 0 1 2 2 2
  line L3343 (-19.4403, 47.7246) -> (-19.6103, 47.7246) construction
  line L3344 (-19.6103, 47.7246) -> (-19.8566, 47.4782) construction
  line L3345 (-19.8566, 47.4782) -> (-19.8566, 47.3082) construction
  line L3346 (-19.8566, 47.3082) -> (-19.8566, 46.0662)
  spline S1048 degree 2 poles (-19.8566, 46.0662) (-19.8566, 45.8962) (-19.6103, 45.6499) (-19.4403, 45.6499) knots 0 0 0 1 2 2 2
  line L3347 (-19.8566, 46.0662) -> (-19.8566, 45.8962) construction
  line L3348 (-19.8566, 45.8962) -> (-19.6103, 45.6499) construction
  line L3349 (-19.6103, 45.6499) -> (-19.4403, 45.6499) construction
  line L3350 (-19.4403, 45.6499) -> (-18.8193, 45.6499)
  spline S1049 degree 2 poles (-18.8193, 45.6499) (-18.6111, 45.6499) (-18.6111, 45.4417) knots 0 0 0 1 1 1
  line L3351 (-18.8193, 45.6499) -> (-18.6111, 45.6499) construction
  line L3352 (-18.6111, 45.6499) -> (-18.6111, 45.4417) construction
  spline S1050 degree 2 poles (-18.6111, 45.4417) (-18.6111, 45.2336) (-18.8193, 45.2336) knots 0 0 0 1 1 1
  line L3353 (-18.6111, 45.4417) -> (-18.6111, 45.2336) construction
  line L3354 (-18.6111, 45.2336) -> (-18.8193, 45.2336) construction
  line L3355 (-18.8193, 45.2336) -> (-19.4403, 45.2336)
  spline S1051 degree 2 poles (-14.0455, 47.7246) (-14.2397, 47.7246) (-14.4583, 47.4817) (-14.4583, 47.3117) knots 0 0 0 1 2 2 2
  line L3356 (-14.0455, 47.7246) -> (-14.2397, 47.7246) construction
  line L3357 (-14.2397, 47.7246) -> (-14.4583, 47.4817) construction
  line L3358 (-14.4583, 47.4817) -> (-14.4583, 47.3117) construction
  spline S1052 degree 2 poles (-14.4583, 47.3117) (-14.4583, 47.1417) (-14.3542, 47.0238) knots 0 0 0 1 1 1
  line L3359 (-14.4583, 47.3117) -> (-14.4583, 47.1417) construction
  line L3360 (-14.4583, 47.1417) -> (-14.3542, 47.0238) construction
  spline S1053 degree 2 poles (-14.3542, 47.0238) (-14.2397, 46.8954) (-14.0455, 46.8954) knots 0 0 0 1 1 1
  line L3361 (-14.3542, 47.0238) -> (-14.2397, 46.8954) construction
  line L3362 (-14.2397, 46.8954) -> (-14.0455, 46.8954) construction
  spline S1054 degree 2 poles (-14.493, 45.3273) (-14.5554, 45.2301) (-14.6595, 45.2301) knots 0 0 0 1 1 1
  line L3363 (-14.493, 45.3273) -> (-14.5554, 45.2301) construction
  line L3364 (-14.5554, 45.2301) -> (-14.6595, 45.2301) construction
  spline S1055 degree 2 poles (-14.6595, 45.2301) (-14.7463, 45.2301) (-14.8781, 45.355) (-14.8781, 45.4383) knots 0 0 0 1 2 2 2
  line L3365 (-14.6595, 45.2301) -> (-14.7463, 45.2301) construction
  line L3366 (-14.7463, 45.2301) -> (-14.8781, 45.355) construction
  line L3367 (-14.8781, 45.355) -> (-14.8781, 45.4383) construction
  spline S1056 degree 2 poles (-14.8781, 45.4383) (-14.8781, 45.5007) (-14.8399, 45.5562) knots 0 0 0 1 1 1
  line L3368 (-14.8781, 45.4383) -> (-14.8781, 45.5007) construction
  line L3369 (-14.8781, 45.5007) -> (-14.8399, 45.5562) construction
  line L3370 (-14.8399, 45.5562) -> (-14.2155, 46.493)
  spline S1057 degree 2 poles (-14.2155, 46.493) (-14.5277, 46.545) (-14.7116, 46.7913) knots 0 0 0 1 1 1
  line L3371 (-14.2155, 46.493) -> (-14.5277, 46.545) construction
  line L3372 (-14.5277, 46.545) -> (-14.7116, 46.7913) construction
  spline S1058 degree 2 poles (-14.7116, 46.7913) (-14.8746, 47.0134) (-14.8746, 47.3117) knots 0 0 0 1 1 1
  line L3373 (-14.7116, 46.7913) -> (-14.8746, 47.0134) construction
  line L3374 (-14.8746, 47.0134) -> (-14.8746, 47.3117) construction
  spline S1059 degree 2 poles (-14.8746, 47.3117) (-14.8746, 47.6482) (-14.6665, 47.8807) knots 0 0 0 1 1 1
  line L3375 (-14.8746, 47.3117) -> (-14.8746, 47.6482) construction
  line L3376 (-14.8746, 47.6482) -> (-14.6665, 47.8807) construction
  spline S1060 degree 2 poles (-14.6665, 47.8807) (-14.4375, 48.1409) (-14.0455, 48.1409) knots 0 0 0 1 1 1
  line L3377 (-14.6665, 47.8807) -> (-14.4375, 48.1409) construction
  line L3378 (-14.4375, 48.1409) -> (-14.0455, 48.1409) construction
  line L3379 (-14.0455, 48.1409) -> (-13.0081, 48.1409)
  spline S1061 degree 2 poles (-13.0081, 48.1409) (-12.8, 48.1409) (-12.8, 47.9327) knots 0 0 0 1 1 1
  line L3380 (-13.0081, 48.1409) -> (-12.8, 48.1409) construction
  line L3381 (-12.8, 48.1409) -> (-12.8, 47.9327) construction
  line L3382 (-12.8, 47.9327) -> (-12.8, 45.4417)
  spline S1062 degree 2 poles (-12.8, 45.4417) (-12.8, 45.2336) (-13.0081, 45.2336) knots 0 0 0 1 1 1
  line L3383 (-12.8, 45.4417) -> (-12.8, 45.2336) construction
  line L3384 (-12.8, 45.2336) -> (-13.0081, 45.2336) construction
  spline S1063 degree 2 poles (-13.0081, 45.2336) (-13.2163, 45.2336) (-13.2163, 45.4417) knots 0 0 0 1 1 1
  line L3385 (-13.0081, 45.2336) -> (-13.2163, 45.2336) construction
  line L3386 (-13.2163, 45.2336) -> (-13.2163, 45.4417) construction
  spline S1064 degree 2 poles (-11.1382, 46.4791) (-11.3463, 46.4791) (-11.3463, 46.6872) knots 0 0 0 1 1 1
  line L3387 (-11.1382, 46.4791) -> (-11.3463, 46.4791) construction
  line L3388 (-11.3463, 46.4791) -> (-11.3463, 46.6872) construction
  spline S1065 degree 2 poles (-11.3463, 46.6872) (-11.3463, 46.8954) (-11.1382, 46.8954) knots 0 0 0 1 1 1
  line L3389 (-11.3463, 46.6872) -> (-11.3463, 46.8954) construction
  line L3390 (-11.3463, 46.8954) -> (-11.1382, 46.8954) construction
  line L3391 (-11.1382, 46.8954) -> (-10.93, 46.8954)
  spline S1066 degree 2 poles (-10.93, 46.8954) (-10.7357, 46.8954) (-10.6212, 47.0238) knots 0 0 0 1 1 1
  line L3392 (-10.93, 46.8954) -> (-10.7357, 46.8954) construction
  line L3393 (-10.7357, 46.8954) -> (-10.6212, 47.0238) construction
  spline S1067 degree 2 poles (-10.6212, 47.0238) (-10.5171, 47.1417) (-10.5171, 47.3117) knots 0 0 0 1 1 1
  line L3394 (-10.6212, 47.0238) -> (-10.5171, 47.1417) construction
  line L3395 (-10.5171, 47.1417) -> (-10.5171, 47.3117) construction
  spline S1068 degree 2 poles (-10.5171, 47.3117) (-10.5171, 47.4817) (-10.6212, 47.5962) knots 0 0 0 1 1 1
  line L3396 (-10.5171, 47.3117) -> (-10.5171, 47.4817) construction
  line L3397 (-10.5171, 47.4817) -> (-10.6212, 47.5962) construction
  spline S1069 degree 2 poles (-10.6212, 47.5962) (-10.7357, 47.7246) (-10.9335, 47.7246) knots 0 0 0 1 1 1
  line L3398 (-10.6212, 47.5962) -> (-10.7357, 47.7246) construction
  line L3399 (-10.7357, 47.7246) -> (-10.9335, 47.7246) construction
  line L3400 (-10.9335, 47.7246) -> (-11.1416, 47.7246)
  spline S1070 degree 2 poles (-11.1416, 47.7246) (-11.4226, 47.7246) (-11.6377, 47.558) knots 0 0 0 1 1 1
  line L3401 (-11.1416, 47.7246) -> (-11.4226, 47.7246) construction
  line L3402 (-11.4226, 47.7246) -> (-11.6377, 47.558) construction
  spline S1071 degree 2 poles (-11.6377, 47.558) (-11.7002, 47.5129) (-11.7661, 47.5129) knots 0 0 0 1 1 1
  line L3403 (-11.6377, 47.558) -> (-11.7002, 47.5129) construction
  line L3404 (-11.7002, 47.5129) -> (-11.7661, 47.5129) construction
  spline S1072 degree 2 poles (-11.7661, 47.5129) (-11.8494, 47.5129) (-11.9743, 47.6413) (-11.9743, 47.728) knots 0 0 0 1 2 2 2
  line L3405 (-11.7661, 47.5129) -> (-11.8494, 47.5129) construction
  line L3406 (-11.8494, 47.5129) -> (-11.9743, 47.6413) construction
  line L3407 (-11.9743, 47.6413) -> (-11.9743, 47.728) construction
  spline S1073 degree 2 poles (-11.9743, 47.728) (-11.9743, 47.8252) (-11.8875, 47.8911) knots 0 0 0 1 1 1
  line L3408 (-11.9743, 47.728) -> (-11.9743, 47.8252) construction
  line L3409 (-11.9743, 47.8252) -> (-11.8875, 47.8911) construction
  spline S1074 degree 2 poles (-11.8875, 47.8911) (-11.5649, 48.1409) (-11.1416, 48.1409) knots 0 0 0 1 1 1
  line L3410 (-11.8875, 47.8911) -> (-11.5649, 48.1409) construction
  line L3411 (-11.5649, 48.1409) -> (-11.1416, 48.1409) construction
  line L3412 (-11.1416, 48.1409) -> (-10.9335, 48.1409)
  spline S1075 degree 2 poles (-10.9335, 48.1409) (-10.5414, 48.1409) (-10.309, 47.8842) knots 0 0 0 1 1 1
  line L3413 (-10.9335, 48.1409) -> (-10.5414, 48.1409) construction
  line L3414 (-10.5414, 48.1409) -> (-10.309, 47.8842) construction
  spline S1076 degree 2 poles (-10.309, 47.8842) (-10.1008, 47.6482) (-10.1008, 47.3117) knots 0 0 0 1 1 1
  line L3415 (-10.309, 47.8842) -> (-10.1008, 47.6482) construction
  line L3416 (-10.1008, 47.6482) -> (-10.1008, 47.3117) construction
  spline S1077 degree 2 poles (-10.1008, 47.3117) (-10.1008, 46.9266) (-10.361, 46.6872) knots 0 0 0 1 1 1
  line L3417 (-10.1008, 47.3117) -> (-10.1008, 46.9266) construction
  line L3418 (-10.1008, 46.9266) -> (-10.361, 46.6872) construction
  spline S1078 degree 2 poles (-10.361, 46.6872) (-10.1008, 46.4479) (-10.1008, 46.0628) knots 0 0 0 1 1 1
  line L3419 (-10.361, 46.6872) -> (-10.1008, 46.4479) construction
  line L3420 (-10.1008, 46.4479) -> (-10.1008, 46.0628) construction
  spline S1079 degree 2 poles (-10.1008, 46.0628) (-10.1008, 45.7228) (-10.309, 45.4903) knots 0 0 0 1 1 1
  line L3421 (-10.1008, 46.0628) -> (-10.1008, 45.7228) construction
  line L3422 (-10.1008, 45.7228) -> (-10.309, 45.4903) construction
  spline S1080 degree 2 poles (-10.309, 45.4903) (-10.5414, 45.2336) (-10.9335, 45.2336) knots 0 0 0 1 1 1
  line L3423 (-10.309, 45.4903) -> (-10.5414, 45.2336) construction
  line L3424 (-10.5414, 45.2336) -> (-10.9335, 45.2336) construction
  line L3425 (-10.9335, 45.2336) -> (-11.1416, 45.2336)
  spline S1081 degree 2 poles (-11.1416, 45.2336) (-11.5649, 45.2336) (-11.8875, 45.4834) knots 0 0 0 1 1 1
  line L3426 (-11.1416, 45.2336) -> (-11.5649, 45.2336) construction
  line L3427 (-11.5649, 45.2336) -> (-11.8875, 45.4834) construction
  spline S1082 degree 2 poles (-11.8875, 45.4834) (-11.9743, 45.5493) (-11.9743, 45.6464) knots 0 0 0 1 1 1
  line L3428 (-11.8875, 45.4834) -> (-11.9743, 45.5493) construction
  line L3429 (-11.9743, 45.5493) -> (-11.9743, 45.6464) construction
  spline S1083 degree 2 poles (-11.9743, 45.6464) (-11.9743, 45.7332) (-11.8494, 45.8615) (-11.7661, 45.8615) knots 0 0 0 1 2 2 2
  line L3430 (-11.9743, 45.6464) -> (-11.9743, 45.7332) construction
  line L3431 (-11.9743, 45.7332) -> (-11.8494, 45.8615) construction
  line L3432 (-11.8494, 45.8615) -> (-11.7661, 45.8615) construction
  spline S1084 degree 2 poles (-11.7661, 45.8615) (-11.7002, 45.8615) (-11.6377, 45.8164) knots 0 0 0 1 1 1
  line L3433 (-11.7661, 45.8615) -> (-11.7002, 45.8615) construction
  line L3434 (-11.7002, 45.8615) -> (-11.6377, 45.8164) construction
  spline S1085 degree 2 poles (-11.6377, 45.8164) (-11.4226, 45.6499) (-11.1416, 45.6499) knots 0 0 0 1 1 1
  line L3435 (-11.6377, 45.8164) -> (-11.4226, 45.6499) construction
  line L3436 (-11.4226, 45.6499) -> (-11.1416, 45.6499) construction
  line L3437 (-11.1416, 45.6499) -> (-10.9335, 45.6499)
  spline S1086 degree 2 poles (-10.9335, 45.6499) (-10.7357, 45.6499) (-10.6212, 45.7817) knots 0 0 0 1 1 1